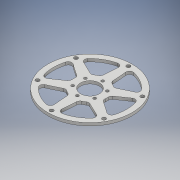
# Autodesk Inventor part: SprocketHubPlate_plasmacut
Saved by Autodesk Inventor 2019.3 (Build 233278000, 278)
## iProperties
Created: 2017-05-06
Part Number: SprocketHubPlate_plasmacut
Material: Generic
Document SubType Name: Modeling
Designer: eroldan
Density: 1 g/cm^3
Appearance: Default
Author: eroldan
Autodesk Inventor part; units mm, degrees
ref_plane "YZ Plane" through (0, 0, 0) normal (1, 0, 0) x (0, 1, 0)
ref_plane "XZ Plane" through (0, 0, 0) normal (0, 1, 0) x (-1, 0, 0)
ref_plane "XY Plane" through (0, 0, 0) normal (0, 0, 1) x (1, 0, 0)
sketch "Sketch1" plane through (0, 0, 0) normal (0, 0, 1) x (1, 0, 0)
  circle A0 centre (0, 0) radius 16.5
  circle A1 centre (0, 0) radius 73
  point P0 (0, 66.675)
  point P1 (-57.7422, 33.3375)
  point P2 (-57.7422, -33.3375)
  point P3 (0, -66.675)
  point P4 (57.7422, -33.3375)
  point P5 (57.7422, 33.3375)
  point P6 (0, 22)
  point P7 (-19.0526, 11)
  point P8 (-19.0526, -11)
  point P9 (0, -22)
  point P10 (19.0526, -11)
  point P11 (19.0526, 11)
  dimension "d0" = 66.675
  dimension "d3" = 360
  dimension "d9" = 33
  dimension "d20" = 22
  dimension "d23" = 360
  dimension "d25" = 146
  constraints: 2 centre point, 1 coincident, 14 other
  measures "d0" distance of point (0, 0) point (0, 66.675)
  measures "d9" diameter of A0
  measures "d20" distance of point (0, 22) point (0, 0)
  measures "d25" diameter of A1
extrude "Extrusion2" add sketch "Sketch1" along normal blind 5
hole "Hole2" at (0, 66.675, 0) at (-57.7422, 33.3375, 0) at (-57.7422, -33.3375, 0) at (0, -66.675, 0) at (57.7422, -33.3375, 0) at (57.7422, 33.3375, 0) direction (0, 0, 1) diameter 6.5 end through all
hole "Hole3" at (0, 22, 0) at (-19.0526, 11, 0) at (-19.0526, -11, 0) at (0, -22, 0) at (19.0526, 11, 0) at (19.0526, -11, 0) direction (0, 0, 1) diameter 5 end through all
sketch "Sketch4" plane through (0, 0, 5) normal (0, 0, 1) x (1, 0, 0)
  circle A0 centre (0, 0) radius 28.9422 construction
  line L0 (0, 0) -> (58.5803, 0) construction
  circle A1 centre (-57.7422, 33.3375) radius 3.25 construction
  circle A2 centre (0, 66.675) radius 3.25 construction
  line L1 (-57.7422, 33.3375) -> (0, 66.675) construction
  circle A3 centre (0, 0) radius 16.5 construction
  circle A4 centre (-19.0526, 11) radius 2.5 construction
  circle A5 centre (0, 22) radius 2.5 construction
  line L2 (-19.0526, 11) -> (0, 22) construction
  circle A6 centre (0, 0) radius 63.4652 construction
  arc A7 (-6.0622, 63.175) -> (-51.6801, 36.8375) centre (0, 0) ccw
  line L3 (-9.5263, 16.5) -> (-21.2308, 36.7728) construction
  line L4 (-8.8547, 27.5544) -> (-19.4354, 21.4456) construction
  line L5 (-8.8547, 27.5544) -> (-6.0622, 63.175)
  line L6 (-19.4354, 21.4456) -> (-51.6801, 36.8375)
  arc A8 (-8.8547, 27.5544) -> (-19.4354, 21.4456) centre (0, 0) ccw
  point P0 (-14.1451, 24.5)
  dimension "d60" = 7
  dimension "d61" = 7
  constraints: 14 end point, 4 point on circle, 3 coincident, 3 point on line, 2 centre point, 2 midpoint, 2 perpendicular, 1 horizontal, 7 other
  measures "d60" distance of L1.end L5.end
  measures "d61" distance of L1.start L6.end
extrude "Extrusion4" cut sketch "Sketch4" against normal blind 10
fillet "Fillet1" radius 6 4 edges at (-51.6801, 36.8375, 2.5) (-6.0622, 63.175, 2.5) (-8.8547, 27.5544, 2.5) (-19.4354, 21.4456, 2.5)
pattern_circular "Circular Pattern1" count 6 over 360 about axis through (0, 0, -10) along (0, 0, 1) of "Extrusion4", "Fillet1"
equation "\"d61\" = d60"
